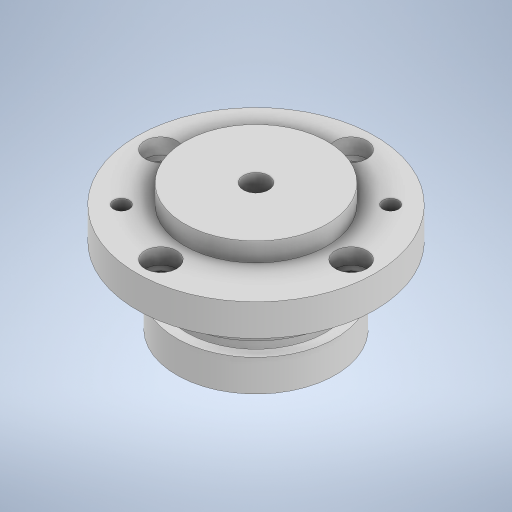
# Autodesk Inventor part: 05-16-2023 Pompa Manuale OLIO
Saved by Autodesk Inventor 2023 (Build 270158000, 158)
## iProperties
Created: 2023-05-16
Part Number: 05-16-2023 Pompa Manuale OLIO
Material: Generico
Document SubType Name: Modeling
Designer: Admin
Density: 1 g/cm^3
Appearance: Default
Author: Admin
Autodesk Inventor part; units mm, degrees
ref_plane "YZ Plane" through (0, 0, 0) normal (1, 0, 0) x (0, 1, 0)
ref_plane "XZ Plane" through (0, 0, 0) normal (0, 1, 0) x (-1, 0, 0)
ref_plane "XY Plane" through (0, 0, 0) normal (0, 0, 1) x (1, 0, 0)
sketch "Schizzo1" plane through (0, 0, 0) normal (0, 0, 1) x (1, 0, 0)
  line L0 (0, 0) -> (0, 24.2842) construction
  line L1 (-25, 0) -> (-25, 10)
  line L2 (-25, 10) -> (-21.85, 10)
  line L3 (-21.85, 10) -> (-21.85, 14.5)
  line L4 (-21.85, 14.5) -> (-25, 14.5)
  line L5 (-25, 14.5) -> (-25, 24)
  line L6 (-25, 24) -> (-37.5, 24)
  line L7 (-37.5, 24) -> (-37.5, 34)
  line L8 (-37.5, 34) -> (-22.5, 34)
  line L9 (-22.5, 34) -> (-22.5, 40)
  line L10 (-22.5, 40) -> (-4, 40)
  line L11 (-4, 40) -> (-4, 32)
  line L12 (-4, 32) -> (-15, 32)
  line L13 (-15, 32) -> (-15, 0)
  line L14 (-25, 0) -> (-15, 0)
  dimension "d0" = 30
  dimension "d1" = 8
  dimension "d2" = 43.7
  dimension "d3" = 50
  dimension "d4" = 45
  dimension "d5" = 75
  dimension "d9" = 24
  dimension "d10" = 34
  dimension "d11" = 32
  dimension "d13" = 4.5
  dimension "d14" = 10
  dimension "d15" = 40
  constraints: 30 end point, 12 perpendicular, 2 point on line, 2 vertical, 1 horizontal alignment
  measures "d0" diameter of L13 L0
  measures "d1" diameter of L11 L0
  measures "d2" diameter of L3 L0
  measures "d3" diameter of L5 L0
  measures "d4" diameter of L9 L0
  measures "d5" diameter of L7 L0
  measures "d9" distance between parallel lines of L14 L6
  measures "d10" distance between parallel lines of L14 L8
  measures "d11" distance between parallel lines of L14 L12
  measures "d13" distance between parallel lines of L2 L4
  measures "d14" distance between parallel lines of L14 L2
  measures "d15" distance between parallel lines of L14 L10
revolve "Rivoluzione1" add sketch "Schizzo1" angle 360 about axis through (0, 0, 0) along (0, 1, 0)
sketch "Schizzo2" plane through (0, 34, 0) normal (0, 1, 0) x (1, 0, 0)
  circle A0 centre (0, 0) radius 25 projected
  circle A1 centre (0, 0) radius 30 construction
  circle A2 centre (30, 0) radius 3.496
  circle A3 centre (0, 30) radius 2.9704
  circle A4 centre (-30, 0) radius 3.7285
  circle A5 centre (0, -30) radius 3.043
  circle A6 centre (-21.2132, -21.2132) radius 2.9112
  circle A7 centre (21.2132, 21.2132) radius 2.3494
  dimension "d17" = 60
  dimension "d18" = 45
  dimension "d19" = 45
  constraints: 7 centre point, 6 point on circle, 1 coincident
  measures "d17" diameter of A1
hole "Foro1" at (-30, 34, 0) at (0, 34, -30) at (30, 34, 0) at (0, 34, 30) direction (0, -1, 0) diameter 5.5 end through all counterbore diameter 10 counterbore depth 5
hole "Foro2" at (21.2132, 34, -21.2132) at (-21.2132, 34, 21.2132) direction (0, -1, 0) diameter 5 end through all
